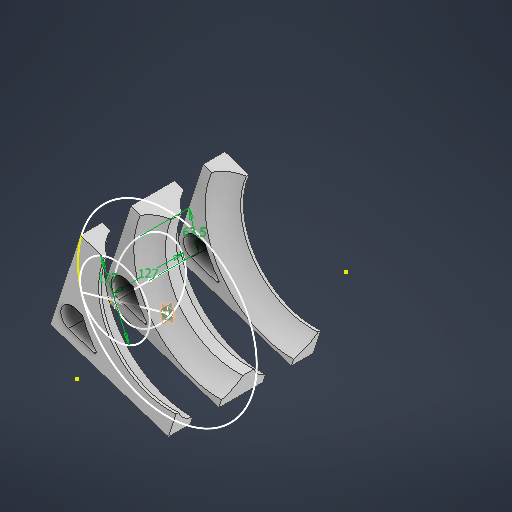
# Autodesk Inventor part: траектория 25-26
Saved by Autodesk Inventor 2025 (Build 290162000, 162)
## iProperties
Created: 2025-10-03
Part Number: траектория 25-26
Material: Типовые
Document SubType Name: Modeling
Designer: Phantom
Density: 1 g/cm^3
Appearance: По умолчанию
Author: Phantom
Autodesk Inventor part; units mm, degrees
sketch "Эскиз1" plane through (0, 0, 0) normal (0, 0, 1) x (1, 0, 0)
  line L0 (14.5513, 220.3235) -> (16.6686, 220.3036)
  line L1 (220, 0) -> (230, 0) construction
  line L2 (0, 0) -> (170, 0)
  line L3 (170, 0) -> (170, 2)
  arc A0 (14.5513, 220.3235) -> (170, 0) centre (170, 165) ccw
  arc A1 (16.6686, 220.3036) -> (170, 2) centre (170, 165) ccw
  line L4 (170, 1) -> (170, 0)
  dimension "d12" = 330
  dimension "d13" = 2
  constraints: 10 end point, 4 point on circle, 2 centre point, 2 horizontal, 1 midpoint, 1 vertical
  measures "d12" diameter of A0
  measures "d13" radial gap between concentric circles of A0 A1
extrude "Выдавливание1" add sketch "Эскиз1" along normal blind 385
sketch "Эскиз2" plane through (0, 0, 0) normal (0, 0, -1) x (-1, 0, 0)
  line L0 (-16.6686, 220.3036) -> (-14.5513, 220.3235) projected
  arc A0 (-170, 2) -> (-16.6686, 220.3036) centre (-170, 165) ccw projected
  line L1 (-170, 0) -> (-170, 2) projected
  arc A1 (-170, 0) -> (-14.5513, 220.3235) centre (-170, 165) ccw projected
  point P0 (0, 0)
extrude "Выдавливание2" cut sketch "Эскиз2" against normal blind 121
chamfer "Фаска1" distance 2 angle 45 1 edges at (170, 2, 253)
chamfer "Фаска2" distance 2.8 angle 45 1 edges at (168.0001, 2.0123, 253)
sketch "Эскиз4" plane through (0, 0, 385) normal (0, 0, 1) x (1, 0, 0)
  line L0 (165.2006, 2.0707) -> (169.9739, 0.0263) projected
  arc A0 (16.6686, 220.3036) -> (165.2006, 2.0707) centre (170, 165) ccw projected
  line L1 (16.6686, 220.3036) -> (14.5513, 220.3235) projected
  arc A1 (14.5513, 220.3235) -> (170, 0) centre (170, 165) ccw projected
  line L2 (169.9739, 0.0263) -> (170, 0) projected
  arc A2 (8.48, 230.7703) -> (172.1929, 23.6823) centre (165.364, 186.5392) ccw projected
  arc A3 (6.3666, 230.6392) -> (177.1276, 21.959) centre (165.364, 186.5392) ccw projected
  line L3 (8.48, 230.7703) -> (6.3666, 230.6392) projected
  point P0 (0, 0)
  point P1 (6.736, 141.1283)
  point P2 (5.2437, 156.0352)
extrude "Выдавливание3" add sketch "Эскиз4" against normal up to surface (264 mm away) contours A3 L3 A2 A1
sketch "Эскиз5" plane through (0, 0, 385) normal (0, 0, 1) x (1, 0, 0)
  point P0 (0, 0)
sketch "Эскиз6" plane through (0, 0, 385) normal (0, 0, 1) x (1, 0, 0)
  arc A0 (8.48, 230.7703) -> (172.1929, 23.6823) centre (165.364, 186.5392) ccw projected
  arc A1 (4.2174, 151.0884) -> (177.1276, 21.959) centre (165.364, 186.5392) ccw projected
  arc A2 (6.3666, 230.6392) -> (6.736, 141.1283) centre (165.364, 186.5392) ccw projected
  line L0 (8.48, 230.7703) -> (6.3666, 230.6392) projected
  line L1 (165.2006, 2.0707) -> (169.9739, 0.0263) projected
  arc A3 (16.6686, 220.3036) -> (165.2006, 2.0707) centre (170, 165) ccw projected
  line L2 (16.6686, 220.3036) -> (14.5513, 220.3235) projected
  arc A4 (14.5513, 220.3235) -> (5.2437, 156.0352) centre (170, 165) ccw projected
  arc A5 (8.48, 230.7703) -> (5.2437, 156.0352) centre (165.364, 186.5392) ccw projected
  line L3 (8.48, 230.7703) -> (6.3666, 230.6392) projected
  arc A6 (6.3666, 230.6392) -> (6.736, 141.1283) centre (165.364, 186.5392) ccw projected
  arc A7 (6.736, 141.1283) -> (170, 0) centre (170, 165) ccw projected
  line L4 (169.9739, 0.0263) -> (170, 0) projected
  point P0 (0, 0)
  point P1 (5.2437, 156.0352)
  point P2 (8.6956, 141.5501)
extrude "Выдавливание4" cut sketch "Эскиз6" against normal through all contours A4 L2 A3 A0
sketch "Эскиз7" plane through (0, 0, 385) normal (0, 0, 1) x (1, 0, 0)
  arc A0 (8.48, 230.7703) -> (8.6956, 141.5501) centre (165.364, 186.5392) ccw projected
  line L0 (8.48, 230.7703) -> (6.3666, 230.6392) projected
  arc A1 (6.3666, 230.6392) -> (6.736, 141.1283) centre (165.364, 186.5392) ccw projected
  arc A2 (6.736, 141.1283) -> (170, 0) centre (170, 165) ccw projected
  line L1 (169.9739, 0.0263) -> (170, 0) projected
  line L2 (165.2006, 2.0707) -> (169.9739, 0.0263) projected
  arc A3 (8.6956, 141.5501) -> (165.2006, 2.0707) centre (170, 165) ccw projected
  line L3 (7.9507, 133.9351) -> (-40.0993, 149.5316)
  line L4 (-49.858, 62.7801) -> (67.4599, 424.2168) projected
  line L5 (-49.858, 62.7801) -> (127.0544, 5.6869)
  line L6 (-49.858, 62.7801) -> (-48.0056, 68.487)
  line L7 (-48.0056, 68.487) -> (101.3216, 20.2961)
  line L8 (86.2538, 25.1587) -> (84.4111, 19.4487)
  line L9 (-13.7205, 69.3639) -> (64.1078, 44.2472)
  line L10 (-13.7205, 69.3639) -> (-53.2073, 82.1071)
  line L11 (6.3666, 230.6392) -> (-61.8212, 20.5641)
  line L12 (0.3654, 112.7603) -> (33.0364, 102.1557)
  line L13 (0.3654, 112.7603) -> (-39.1966, 125.6017)
  point P0 (0, 0)
  point P1 (-42.9225, 78.788)
  point P2 (-48.2834, 62.2719)
  point P3 (85.6236, 23.2057)
  point P4 (54.2251, 47.4365)
  point P5 (-21.8795, 143.6177)
  point P6 (-28.8205, 122.2337)
  point P7 (15.1754, 107.9532)
  dimension "d24" = 6
  constraints: 20 end point, 4 parallel, 3 point on circle, 3 point on line, 2 perpendicular, 1 collinear, 2 other
  measures "d24" distance of L4.start L6.end
extrude "Выдавливание5" add sketch "Эскиз7" against normal up to surface (264 mm away) contours A1 A2 L3 L11 | L3 A2 L12 L13 L11 | A2 L7 L11 L10 L9 | A2 L8 L5 L11 L7
sketch "Эскиз8" plane through (0, 0, 385) normal (0, 0, 1) x (1, 0, 0)
  arc A0 (-12.5279, 69.512) -> (1.2437, 111.9401) centre (-8.4636, 91.6419) ccw projected
  arc A1 (15.1754, 107.9532) -> (54.2251, 47.4365) centre (170, 165) ccw projected
  arc A2 (9.1771, 109.9002) -> (50.7168, 43.874) centre (170, 165) ccw
  line L0 (-28.8205, 122.2337) -> (15.1754, 107.9532) projected
  line L1 (54.2251, 47.4365) -> (-42.9225, 78.788) projected
  point P0 (0, 0)
  point P1 (44.1807, 50.678)
  dimension "d27" = 5
  constraints: 2 point on circle, 1 centre point, 1 point on line
  measures "d27" radial gap between concentric circles of A1 A2
extrude "Выдавливание6" add sketch "Эскиз8" against normal up to surface (264 mm away)
sketch "Эскиз9" plane through (0, 0, 385) normal (0, 0, 1) x (1, 0, 0)
  arc A0 (8.48, 230.7703) -> (8.6956, 141.5501) centre (165.364, 186.5392) ccw projected
  line L0 (8.48, 230.7703) -> (6.3666, 230.6392) projected
  line L1 (6.3666, 230.6392) -> (-28.8205, 122.2337) projected
  line L2 (-28.8205, 122.2337) -> (9.1771, 109.9002) projected
  arc A1 (9.1771, 109.9002) -> (44.1807, 50.678) centre (170, 165) ccw projected
  line L3 (44.1807, 50.678) -> (-42.9225, 78.788) projected
  line L4 (-42.9225, 78.788) -> (-48.2834, 62.2719) projected
  line L5 (-48.2834, 62.2719) -> (84.4111, 19.4487) projected
  line L6 (84.4111, 19.4487) -> (85.6236, 23.2057) projected
  arc A2 (85.6236, 23.2057) -> (170, 0) centre (170, 165) ccw projected
  line L7 (169.9739, 0.0263) -> (170, 0) projected
  line L8 (165.2006, 2.0707) -> (169.9739, 0.0263) projected
  arc A3 (8.6956, 141.5501) -> (165.2006, 2.0707) centre (170, 165) ccw projected
  line L9 (85.6236, 23.2057) -> (90.4504, 38.1623)
  line L10 (84.4111, 19.4487) -> (85.6236, 23.2057) projected
  point P0 (0, 0)
  point P1 (86.2538, 25.1587)
  constraints: 2 end point, 1 collinear
extrude "Выдавливание7" cut sketch "Эскиз9" against normal through all contours A3 L8 L7 A2 L9
sketch "Эскиз10" plane through (0, 0, 385) normal (0, 0, 1) x (1, 0, 0)
  line L0 (8.48, 230.7703) -> (6.3666, 230.6392) projected
  line L1 (-48.2834, 62.2719) -> (6.3666, 230.6392)
  line L2 (-48.2834, 62.2719) -> (96.336, 15.3303)
  line L3 (84.4111, 19.4487) -> (86.2538, 25.1587) projected
  arc A0 (8.6956, 141.5501) -> (86.2538, 25.1587) centre (170, 165) ccw projected
  arc A1 (8.48, 230.7703) -> (8.6956, 141.5501) centre (165.364, 186.5392) ccw projected
  line L4 (8.48, 230.7703) -> (6.3666, 230.6392) projected
  line L5 (6.3666, 230.6392) -> (-28.8205, 122.2337) projected
  line L6 (-28.8205, 122.2337) -> (9.1771, 109.9002) projected
  arc A2 (9.1771, 109.9002) -> (44.1807, 50.678) centre (170, 165) ccw projected
  line L7 (44.1807, 50.678) -> (-42.9225, 78.788) projected
  line L8 (-42.9225, 78.788) -> (-48.2834, 62.2719) projected
  line L9 (-48.2834, 62.2719) -> (84.4111, 19.4487) projected
  line L10 (84.4111, 19.4487) -> (83.7893, 17.522)
  line L11 (84.4111, 19.4487) -> (86.2538, 25.1587) projected
  point P0 (0, 0)
  point P1 (84.3387, 19.2244)
  constraints: 6 end point, 1 collinear, 1 perpendicular
extrude "Выдавливание8" add sketch "Эскиз10" against normal up to surface (264 mm away) contours L10 L2 L9
sketch "Эскиз13" plane through (0, 0, 121) normal (0, 0, -1) x (-1, 0, 0)
  arc A0 (18.116, 75.0583) -> (12.6723, 73.0313) centre (8.93, 91.404) ccw projected
  arc A1 (15.1818, 72.1432) -> (12.9717, 71.5614) centre (8.93, 91.404) ccw
  line L0 (8.93, 91.404) -> (31.1796, 22.8568)
  line L1 (42.9225, 78.788) -> (48.2834, 62.2719) projected
  line L2 (8.93, 91.404) -> (-2.0706, 125.2951)
  line L3 (28.8205, 122.2337) -> (-9.1771, 109.9002) projected
  line L4 (-44.1807, 50.678) -> (42.9225, 78.788) projected
  line L5 (-6.3666, 230.6392) -> (28.8205, 122.2337) projected
  line L6 (28.8205, 122.2337) -> (42.9225, 78.788)
  line L7 (-27.6965, 100.8055) -> (34.3413, 120.9422)
  line L8 (-44.935, 52.7423) -> (51.7275, 83.9372)
  arc A2 (-44.1807, 50.678) -> (-9.1771, 109.9002) centre (-170, 165) ccw projected
  point P0 (0, 0)
  point P1 (1.7728, 113.4543)
  point P2 (2.6782, 110.6648)
  point P3 (15.8599, 70.0544)
  point P4 (-10.4135, 106.4154)
  point P5 (2.6782, 110.6648)
  point P6 (-41.3188, 53.9093)
  point P7 (15.1818, 72.1432)
  dimension "d40" = 1.5
  constraints: 10 end point, 3 parallel, 2 point on circle, 2 tangent, 1 centre point, 1 point on line
  measures "d40" radial gap between concentric circles of A0 A1
ref_plane "РабПлоскость1" through (-48.2834, -7.7133, 385) normal (0, 0, -1) x (0.3087313, 0.9511493, 0)
extrude "Выдавливание11" add sketch "Эскиз13" against normal up to surface (264 mm away) contours L8 L6 L4 L0 | L0 L4 A2 L8 | A1 L7 L6 L8 | L7 A2 L3 L2 | L2 L3 L6 L7
fillet "Сопряжение1" radius 3 2 edges at (41.3188, 53.9093, 253) (10.4135, 106.4154, 253)
sketch "Эскиз14" plane through (0, 0, 385) normal (0, 0, 1) x (1, 0, 0)
  line L0 (8.48, 230.7703) -> (6.3666, 230.6392) projected
  line L1 (6.3666, 230.6392) -> (55.6278, 214.6497)
  line L2 (-48.2834, 62.2719) -> (84.3387, 19.2244) projected
  arc A0 (8.48, 230.7703) -> (8.6956, 141.5501) centre (165.364, 186.5392) ccw projected
  point P0 (0, 0)
  point P1 (8.2707, 230.0212)
  constraints: 2 end point, 1 parallel
extrude "Выдавливание12" cut sketch "Эскиз14" against normal through all
sketch "Эскиз15" plane through (6.3666, 230.6392, 385) normal (0.3087313, 0.9511493, 0) x (0.9511493, -0.3087313, 0)
  line L0 (139.423, 0) -> (29.7199, 0) projected
  line L1 (139.423, 264) -> (29.7199, 264) projected
  line L2 (77.6819, 264) -> (77.6819, 0) projected
  line L3 (28.4369, 264) -> (28.4369, 0) projected
  line L4 (0, 264) -> (139.4335, 264) projected
  line L5 (139.4335, 0) -> (139.4335, 264) projected
  line L6 (0, 0) -> (139.4335, 0) projected
  line L7 (0, 0) -> (0, 264) projected
  line L8 (0, 0) -> (0, 40)
  line L9 (0, 40) -> (139.4335, 40)
  line L10 (0, 264) -> (0, 224)
  line L11 (0, 224) -> (139.4335, 224)
  line L12 (0, 132) -> (139.4335, 132)
  line L13 (0, 92) -> (139.4335, 92)
  line L14 (0, 172) -> (139.4335, 172)
  line L15 (28.4369, 264) -> (28.4369, 0) projected
  line L16 (28.4369, 92) -> (-4.7788, 92)
  line L17 (28.4369, 132) -> (-6.4168, 132)
  line L18 (28.4369, 172) -> (-6.4168, 172)
  point P0 (65.15, 385)
  point P1 (28.4369, 172)
  point P2 (139.4335, 172)
  point P3 (28.4369, 224)
  point P4 (28.4369, 92)
  point P5 (28.4369, 40)
  point P6 (139.4335, 92)
  point P7 (28.4369, 172)
  point P8 (28.4369, 92)
  dimension "d47" = 40
  dimension "d48" = 40
  dimension "d49" = 40
  dimension "d50" = 40
  constraints: 20 end point, 10 point on line, 3 midpoint, 2 parallel, 2 perpendicular, 1 horizontal
  measures "d47" distance of L6.start L8.end
  measures "d48" distance of L4.start L10.end
  measures "d49" distance between parallel lines of L12 L13
  measures "d50" distance between parallel lines of L12 L14
extrude "Выдавливание13" cut sketch "Эскиз15" against normal through all contours L9 L3 L13 L2 | L2 L13 L5 L9 | L9 L7 L13 L3 | L14 L3 L11 L2 | L2 L11 L5 L14 | L14 L7 L11 L3
sketch "Эскиз16" plane through (0, 0, 121) normal (0, 0, -1) x (-1, 0, 0)
  line L0 (-6.3666, 230.6392) -> (-8.2707, 230.0212) projected
  arc A0 (-8.6956, 141.5501) -> (-8.2707, 230.0212) centre (-165.364, 186.5392) ccw projected
  arc A1 (-86.2538, 25.1587) -> (-8.6956, 141.5501) centre (-170, 165) ccw projected
  line L1 (-86.2538, 25.1587) -> (-84.3387, 19.2244) projected
  line L2 (48.2834, 62.2719) -> (-84.3387, 19.2244) projected
  line L3 (-6.3666, 230.6392) -> (48.2834, 62.2719) projected
  arc A2 (-9.0336, 106.8633) -> (-10.9148, 105.0674) centre (-8.1075, 104.0098) ccw projected
  line L4 (-9.0336, 106.8633) -> (2.6782, 110.6648) projected
  arc A3 (15.1818, 72.1432) -> (2.6782, 110.6648) centre (8.93, 91.404) ccw projected
  line L5 (15.1818, 72.1432) -> (15.1818, 72.1432) projected
  line L6 (15.1818, 72.1432) -> (-31.6832, 57.0189) projected
  arc A4 (-34.9871, 61.6969) -> (-31.6832, 57.0189) centre (-32.6046, 59.8739) ccw projected
  arc A5 (-34.9871, 61.6969) -> (-10.9148, 105.0674) centre (-170, 165) ccw projected
  line L7 (-167.3298, -7.7134) -> (-261.1287, 281.2651)
  line L8 (-6.3666, 230.6392) -> (-234.3444, 156.6405)
  line L9 (-84.3387, 19.2244) -> (-167.3298, -7.7134)
  point P0 (0, 0)
  point P1 (-221.9798, 160.6539)
  dimension "d73" = 226.687
  constraints: 6 end point, 2 parallel
  measures "d73" distance between parallel lines of L3 L7
extrude "Выдавливание14" add sketch "Эскиз16" against normal up to surface (264 mm away) contours A0 A1 L1 L9 L7 L8
sketch "Эскиз17" plane through (0, 0, 385) normal (0, 0, 1) x (1, 0, 0)
  arc A0 (8.2707, 230.0212) -> (8.6956, 141.5501) centre (165.364, 186.5392) ccw projected
  line L0 (165.364, 186.5392) -> (8.6956, 141.5501)
  point P0 (0, 0)
  constraints: 2 end point, 1 coincident
ref_plane "РабПлоскость2" through (165.364, 186.5392, 385) normal (-0.9611557, -0.2760066, 0) x (0.2760066, -0.9611557, 0)
ref_plane "РабПлоскость3" through (165.364, 186.5392, 385) normal (0, 0, 1) x (1, 0, 0)
sketch "Эскиз18" plane through (165.364, 186.5392, 385) normal (0, 0, 1) x (1, 0, 0)
  circle A0 centre (0, 0) radius 163
  line L0 (0, 0) -> (-156.6684, -44.9891) projected
  circle A1 centre (-95.635, -27.4627) radius 63.5
  point P0 (-165.364, -186.5392)
  dimension "d55" = 127
  constraints: 1 centre point, 1 coincident, 1 point on line, 3 other
  measures "d55" diameter of A1
ref_plane "РабПлоскость4" through (69.729, 159.0765, 385) normal (-0.9611557, -0.2760066, 0) x (0.2760066, -0.9611557, 0)
sketch "Эскиз19" plane through (69.729, 159.0765, 385) normal (-0.9611557, -0.2760066, 0) x (0.2760066, -0.9611557, 0)
  line L0 (0, 0) -> (0, -127)
  line L1 (0, -40) -> (0, 0) projected
  ellipse E0 centre (0, -63.5) end of major axis (0, 0) minor radius 63.5
  point P0 (133.6516, -385)
  dimension "d57" = 63.5
  dimension "d56" = 127
  constraints: 2 end point, 2 vertical, 1 midpoint, 1 vertical alignment, 2 other
  measures "d56" distance of L0.start L0.end
ref_plane "РабПлоскость6" through (8.6956, 141.5501, 121) normal (-0.3087313, -0.9511493, 0) x (0.9511493, -0.3087313, 0)
sketch "Эскиз20" plane through (8.6956, 141.5501, 121) normal (-0.3087313, -0.9511493, 0) x (0.9511493, -0.3087313, 0)
  circle A0 centre (62.6409, 200.5) radius 63.5
  line L0 (196.9671, 0) -> (196.9671, 264) projected
  line L1 (196.9671, 132) -> (-88.0095, 132)
  circle A1 centre (62.6409, 63.5) radius 63.5
  line L2 (87.6409, 200.5) -> (87.6409, 175.2953)
  point P0 (35.4301, -121)
  dimension "d58" = 127
  dimension "d72" = 25
  constraints: 4 end point, 2 centre point, 1 coincident, 1 horizontal, 1 midpoint, 1 symmetric about line, 1 vertical, 1 other
  measures "d58" diameter of A0
  measures "d72" distance of A0.centre L2.start
sketch "Эскиз21" plane through (0, 0, 121) normal (0, 0, -1) x (-1, 0, 0)
  arc A0 (-86.2538, 25.1587) -> (-8.6956, 141.5501) centre (-170, 165) ccw projected
  circle A1 centre (-170, 165) radius 163
  point P0 (0, 0)
  constraints: 1 centre point, 1 coincident, 1 concentric
sweep "Сдвиг1" cut profiles "Эскиз20" path "Эскиз21" path curves A1
sketch "Эскиз22" plane through (0, 0, 385) normal (0, 0, 1) x (1, 0, 0)
  arc A0 (69.3261, 210.2034) -> (188.0526, 56.13) centre (170, 165) ccw projected
  arc A1 (69.3261, 210.2034) -> (188.0526, 56.13) centre (170, 165) ccw projected
  line L0 (221.9798, 160.6539) -> (188.0526, 56.13) projected
  line L1 (221.9798, 160.6539) -> (69.3261, 210.2034) projected
  line L2 (69.3261, 210.2034) -> (6.3666, 230.6392) projected
  line L3 (6.3666, 230.6392) -> (-48.2834, 62.2719) projected
  line L4 (-48.2834, 62.2719) -> (167.3298, -7.7134) projected
  line L5 (188.0526, 56.13) -> (167.3298, -7.7134) projected
  point P0 (0, 0)
  point P1 (188.0526, 56.13)
  point P2 (69.3261, 210.2034)
extrude "Выдавливание15" cut sketch "Эскиз22" against normal through all contours L1 L0 A0
sketch "Эскиз23" plane through (167.3298, -7.7134, 293) normal (0.9511493, -0.3087313, 0) x (0, 0, -1)
  line L0 (-92, 0) -> (-52, 0) projected
  line L1 (-92, 0) -> (-52, 0)
  line L2 (172, 177.0146) -> (172, 0) projected
  line L3 (172, 0) -> (132, 0)
  line L4 (132, 0) -> (132, 198.8982)
  line L5 (132, 198.8982) -> (172, 198.8982)
  line L6 (172, 198.8982) -> (172, 0)
  line L7 (-92, 0) -> (-52, 0)
  line L8 (-52, 0) -> (-52, 229.2687)
  line L9 (-52, 229.2687) -> (-92, 229.2687)
  line L10 (-92, 229.2687) -> (-92, 0)
  line L11 (0, 0) -> (80, 0) projected
  line L12 (40, 0) -> (0, 0)
  line L13 (0, 0) -> (0, 235.4738)
  line L14 (0, 235.4738) -> (40, 235.4738)
  line L15 (40, 235.4738) -> (40, 0)
  line L16 (40, 0) -> (80, 0)
  line L17 (80, 0) -> (80, 261.9984)
  line L18 (80, 261.9984) -> (40, 261.9984)
  line L19 (40, 261.9984) -> (40, 0)
  line L20 (172, 198.8982) -> (-211.179, 198.8982)
  line L21 (172, 0) -> (-92, 0)
  point P0 (293, -44.3233)
  point P1 (172, 52.7649)
  point P2 (0, 198.8982)
  point P3 (-52, 198.8982)
  point P4 (132, 198.8982)
  point P5 (80, 198.8982)
  dimension "d63" = 40
  dimension "d64" = 40
  dimension "d65" = 40
  constraints: 38 end point, 9 equal length, 6 horizontal, 4 perpendicular, 1 midpoint
  measures "d63" distance of L4.end L5.end
  measures "d64" distance of L9.end L8.end
  measures "d65" distance of L13.end L14.end
extrude "Выдавливание16" cut sketch "Эскиз23" against normal through all contours L8 L20 L13 L21 | L17 L20 L4 L21
sketch "Эскиз24" plane through (0, 0, 385) normal (0, 0, 1) x (1, 0, 0)
  arc A0 (69.3261, 210.2034) -> (188.0526, 56.13) centre (170, 165) ccw projected
  circle A1 centre (170, 165) radius 130
  point P0 (0, 0)
  point P1 (100.6289, 69.4118)
  point P2 (61.913, 212.6096)
  dimension "d68" = 260
  constraints: 1 centre point, 1 coincident
  measures "d68" diameter of A1
extrude "Выдавливание17" cut sketch "Эскиз24" against normal through all
